Autodesk Fusion 360 part; units mm, degrees
note: some values were not read from the file. Chosen so that the rebuilt part matches the saved one: a direction. Set by a fixed rule: which sketch regions a step uses.
(part 3 of 5)
  spline S34 degree 5 poles (-9.6039, 49.6725) (-9.6022, 49.6779) (-9.5989, 49.6887) (-9.5943, 49.705) (-9.5889, 49.727) (-9.5833, 49.7547) (-9.5784, 49.7827) (-9.574, 49.8108) (-9.5699, 49.8389) (-9.566, 49.8672) (-9.5622, 49.8955) (-9.5587, 49.9238) (-9.5555, 49.9523) (-9.5527, 49.9808) (-9.5502, 50.0094) (-9.5481, 50.0382) (-9.5463, 50.067) (-9.5447, 50.0958) (-9.5434, 50.1247) (-9.5422, 50.1537) (-9.5413, 50.1827) (-9.5406, 50.2117) (-9.5401, 50.2408) (-9.5399, 50.27) (-9.5399, 50.2992) (-9.5401, 50.3285) (-9.5405, 50.3578) (-9.5412, 50.3871) (-9.542, 50.4165) (-9.543, 50.4459) (-9.5442, 50.4754) (-9.5456, 50.5049) (-9.5473, 50.5344) (-9.549, 50.564) (-9.551, 50.5936) (-9.5532, 50.6232) (-9.5556, 50.6529) (-9.5581, 50.6826) (-9.5608, 50.7123) (-9.5637, 50.7421) (-9.5668, 50.7719) (-9.57, 50.8017) (-9.5734, 50.8315) (-9.577, 50.8614) (-9.5807, 50.8913) (-9.5846, 50.9212) (-9.5887, 50.9511) (-9.593, 50.9811) (-9.5974, 51.0111) (-9.6019, 51.0411) (-9.6067, 51.0711) (-9.6116, 51.1012) (-9.6166, 51.1312) (-9.6218, 51.1613) (-9.6272, 51.1914) (-9.6327, 51.2216) (-9.6384, 51.2517) (-9.6442, 51.2818) (-9.6502, 51.312) (-9.6563, 51.3422) (-9.6626, 51.3724) (-9.6691, 51.4026) (-9.6757, 51.4328) (-9.6824, 51.4631) (-9.6893, 51.4933) (-9.6963, 51.5236) (-9.7035, 51.5539) (-9.7108, 51.5841) (-9.7183, 51.6144) (-9.7259, 51.6447) (-9.7337, 51.675) (-9.74, 51.6993) (-9.7448, 51.7175) (-9.748, 51.7296) (-9.7497, 51.7357) knots 0 0 0 0 0 0 0.01428571 0.02857143 0.04285714 0.05714286 0.07142857 0.08571429 0.1 0.11428571 0.12857143 0.14285714 0.15714286 0.17142857 0.18571429 0.2 0.21428571 0.22857143 0.24285714 0.25714286 0.27142857 0.28571429 0.3 0.31428571 0.32857143 0.34285714 0.35714286 0.37142857 0.38571429 0.4 0.41428571 0.42857143 0.44285714 0.45714286 0.47142857 0.48571429 0.5 0.51428571 0.52857143 0.54285714 0.55714286 0.57142857 0.58571429 0.6 0.61428571 0.62857143 0.64285714 0.65714286 0.67142857 0.68571429 0.7 0.71428571 0.72857143 0.74285714 0.75714286 0.77142857 0.78571429 0.8 0.81428571 0.82857143 0.84285714 0.85714286 0.87142857 0.88571429 0.9 0.91428571 0.92857143 0.94285714 0.95714286 0.97142857 0.98571429 1 1 1 1 1 1
  arc A70 (-9.7497, 51.7357) -> (-10.533, 51.9206) centre (-13.5, 37.5997) ccw
  spline S35 degree 5 poles (-10.533, 51.9206) (-10.5372, 51.9159) (-10.5455, 51.9065) (-10.5579, 51.8924) (-10.5744, 51.8735) (-10.5949, 51.8499) (-10.6153, 51.8262) (-10.6355, 51.8024) (-10.6556, 51.7786) (-10.6756, 51.7547) (-10.6954, 51.7308) (-10.7151, 51.7068) (-10.7346, 51.6828) (-10.754, 51.6587) (-10.7733, 51.6346) (-10.7924, 51.6104) (-10.8114, 51.5861) (-10.8303, 51.5618) (-10.849, 51.5375) (-10.8675, 51.513) (-10.8859, 51.4886) (-10.9042, 51.464) (-10.9223, 51.4395) (-10.9403, 51.4148) (-10.9581, 51.3901) (-10.9757, 51.3654) (-10.9933, 51.3406) (-11.0106, 51.3157) (-11.0278, 51.2908) (-11.0448, 51.2659) (-11.0617, 51.2409) (-11.0784, 51.2158) (-11.095, 51.1907) (-11.1114, 51.1655) (-11.1276, 51.1403) (-11.1437, 51.115) (-11.1596, 51.0897) (-11.1753, 51.0643) (-11.1908, 51.0389) (-11.2062, 51.0134) (-11.2214, 50.9879) (-11.2364, 50.9623) (-11.2513, 50.9366) (-11.2659, 50.9109) (-11.2803, 50.8852) (-11.2946, 50.8594) (-11.3087, 50.8335) (-11.3226, 50.8076) (-11.3363, 50.7816) (-11.3498, 50.7556) (-11.363, 50.7296) (-11.3761, 50.7034) (-11.3889, 50.6772) (-11.4015, 50.651) (-11.4139, 50.6247) (-11.426, 50.5983) (-11.4379, 50.5719) (-11.4497, 50.5455) (-11.4612, 50.519) (-11.4724, 50.4924) (-11.4834, 50.4658) (-11.494, 50.4391) (-11.5042, 50.4123) (-11.514, 50.3854) (-11.5236, 50.3585) (-11.5329, 50.3315) (-11.542, 50.3045) (-11.5509, 50.2774) (-11.5595, 50.2503) (-11.5677, 50.2231) (-11.575, 50.1958) (-11.5801, 50.1737) (-11.5833, 50.1571) (-11.5851, 50.1459) (-11.586, 50.1403) knots -1 -1 -1 -1 -1 -1 -0.98571429 -0.97142857 -0.95714286 -0.94285714 -0.92857143 -0.91428571 -0.9 -0.88571429 -0.87142857 -0.85714286 -0.84285714 -0.82857143 -0.81428571 -0.8 -0.78571429 -0.77142857 -0.75714286 -0.74285714 -0.72857143 -0.71428571 -0.7 -0.68571429 -0.67142857 -0.65714286 -0.64285714 -0.62857143 -0.61428571 -0.6 -0.58571429 -0.57142857 -0.55714286 -0.54285714 -0.52857143 -0.51428571 -0.5 -0.48571429 -0.47142857 -0.45714286 -0.44285714 -0.42857143 -0.41428571 -0.4 -0.38571429 -0.37142857 -0.35714286 -0.34285714 -0.32857143 -0.31428571 -0.3 -0.28571429 -0.27142857 -0.25714286 -0.24285714 -0.22857143 -0.21428571 -0.2 -0.18571429 -0.17142857 -0.15714286 -0.14285714 -0.12857143 -0.11428571 -0.1 -0.08571429 -0.07142857 -0.05714286 -0.04285714 -0.02857143 -0.01428571 0 0 0 0 0 0
  line L35 (-11.586, 50.1403) -> (-11.6601, 49.6588)
  arc A71 (-11.7733, 49.5751) -> (-11.6601, 49.6588) centre (-11.759, 49.674) ccw
  arc A72 (-11.7733, 49.5751) -> (-12.7912, 49.6781) centre (-13.5, 37.5997) ccw
  arc A73 (-12.8852, 49.7829) -> (-12.7912, 49.6781) centre (-12.7853, 49.778) ccw
  line L36 (-12.8852, 49.7829) -> (-12.8614, 50.2695)
  spline S36 degree 5 poles (-12.8614, 50.2695) (-12.8611, 50.2751) (-12.8607, 50.2864) (-12.8605, 50.3034) (-12.861, 50.326) (-12.8627, 50.3543) (-12.8652, 50.3825) (-12.8683, 50.4108) (-12.8716, 50.4391) (-12.8751, 50.4674) (-12.8788, 50.4957) (-12.8827, 50.524) (-12.887, 50.5523) (-12.8916, 50.5806) (-12.8967, 50.6089) (-12.902, 50.6372) (-12.9077, 50.6654) (-12.9137, 50.6937) (-12.9199, 50.722) (-12.9263, 50.7502) (-12.9329, 50.7785) (-12.9397, 50.8068) (-12.9468, 50.835) (-12.9541, 50.8632) (-12.9617, 50.8914) (-12.9695, 50.9196) (-12.9775, 50.9478) (-12.9857, 50.976) (-12.9941, 51.0042) (-13.0027, 51.0323) (-13.0115, 51.0605) (-13.0205, 51.0886) (-13.0297, 51.1167) (-13.0391, 51.1448) (-13.0486, 51.1729) (-13.0584, 51.201) (-13.0684, 51.229) (-13.0785, 51.257) (-13.0888, 51.2851) (-13.0993, 51.3131) (-13.11, 51.341) (-13.1208, 51.369) (-13.1318, 51.3969) (-13.143, 51.4249) (-13.1544, 51.4528) (-13.1659, 51.4807) (-13.1776, 51.5085) (-13.1895, 51.5364) (-13.2015, 51.5642) (-13.2137, 51.592) (-13.226, 51.6198) (-13.2385, 51.6475) (-13.2512, 51.6753) (-13.264, 51.703) (-13.277, 51.7307) (-13.2901, 51.7583) (-13.3034, 51.786) (-13.3168, 51.8136) (-13.3304, 51.8412) (-13.3441, 51.8687) (-13.358, 51.8963) (-13.3721, 51.9238) (-13.3862, 51.9513) (-13.4006, 51.9788) (-13.4151, 52.0062) (-13.4297, 52.0336) (-13.4445, 52.061) (-13.4594, 52.0883) (-13.4744, 52.1157) (-13.4896, 52.143) (-13.505, 52.1702) (-13.5173, 52.192) (-13.5267, 52.2084) (-13.533, 52.2192) (-13.5361, 52.2247) knots 0 0 0 0 0 0 0.01428571 0.02857143 0.04285714 0.05714286 0.07142857 0.08571429 0.1 0.11428571 0.12857143 0.14285714 0.15714286 0.17142857 0.18571429 0.2 0.21428571 0.22857143 0.24285714 0.25714286 0.27142857 0.28571429 0.3 0.31428571 0.32857143 0.34285714 0.35714286 0.37142857 0.38571429 0.4 0.41428571 0.42857143 0.44285714 0.45714286 0.47142857 0.48571429 0.5 0.51428571 0.52857143 0.54285714 0.55714286 0.57142857 0.58571429 0.6 0.61428571 0.62857143 0.64285714 0.65714286 0.67142857 0.68571429 0.7 0.71428571 0.72857143 0.74285714 0.75714286 0.77142857 0.78571429 0.8 0.81428571 0.82857143 0.84285714 0.85714286 0.87142857 0.88571429 0.9 0.91428571 0.92857143 0.94285714 0.95714286 0.97142857 0.98571429 1 1 1 1 1 1
  arc A74 (-13.5361, 52.2247) -> (-14.3406, 52.2005) centre (-13.5, 37.5997) ccw
  spline S37 degree 5 poles (-14.3406, 52.2005) (-14.3434, 52.1949) (-14.349, 52.1837) (-14.3574, 52.1668) (-14.3684, 52.1443) (-14.3821, 52.1162) (-14.3957, 52.088) (-14.4091, 52.0598) (-14.4223, 52.0317) (-14.4354, 52.0034) (-14.4484, 51.9752) (-14.4612, 51.9469) (-14.4738, 51.9187) (-14.4863, 51.8904) (-14.4987, 51.8621) (-14.5109, 51.8337) (-14.523, 51.8054) (-14.5349, 51.777) (-14.5466, 51.7487) (-14.5583, 51.7203) (-14.5697, 51.6919) (-14.581, 51.6635) (-14.5921, 51.635) (-14.6031, 51.6066) (-14.6139, 51.5781) (-14.6246, 51.5497) (-14.6351, 51.5212) (-14.6454, 51.4927) (-14.6556, 51.4642) (-14.6656, 51.4357) (-14.6754, 51.4071) (-14.6851, 51.3786) (-14.6946, 51.3501) (-14.7039, 51.3215) (-14.713, 51.2929) (-14.722, 51.2644) (-14.7308, 51.2358) (-14.7394, 51.2072) (-14.7478, 51.1786) (-14.7561, 51.15) (-14.7642, 51.1214) (-14.772, 51.0928) (-14.7797, 51.0642) (-14.7872, 51.0356) (-14.7945, 51.007) (-14.8016, 50.9784) (-14.8085, 50.9497) (-14.8152, 50.9211) (-14.8217, 50.8925) (-14.828, 50.8639) (-14.8341, 50.8353) (-14.8399, 50.8066) (-14.8456, 50.778) (-14.8509, 50.7494) (-14.8561, 50.7208) (-14.861, 50.6922) (-14.8657, 50.6636) (-14.8701, 50.635) (-14.8744, 50.6064) (-14.8784, 50.5779) (-14.8821, 50.5493) (-14.8854, 50.5208) (-14.8883, 50.4923) (-14.8909, 50.4637) (-14.8931, 50.4353) (-14.8951, 50.4068) (-14.8969, 50.3783) (-14.8985, 50.3499) (-14.8999, 50.3215) (-14.9007, 50.2931) (-14.9007, 50.2648) (-14.8999, 50.2422) (-14.8987, 50.2253) (-14.8976, 50.214) (-14.897, 50.2084) knots -1 -1 -1 -1 -1 -1 -0.98571429 -0.97142857 -0.95714286 -0.94285714 -0.92857143 -0.91428571 -0.9 -0.88571429 -0.87142857 -0.85714286 -0.84285714 -0.82857143 -0.81428571 -0.8 -0.78571429 -0.77142857 -0.75714286 -0.74285714 -0.72857143 -0.71428571 -0.7 -0.68571429 -0.67142857 -0.65714286 -0.64285714 -0.62857143 -0.61428571 -0.6 -0.58571429 -0.57142857 -0.55714286 -0.54285714 -0.52857143 -0.51428571 -0.5 -0.48571429 -0.47142857 -0.45714286 -0.44285714 -0.42857143 -0.41428571 -0.4 -0.38571429 -0.37142857 -0.35714286 -0.34285714 -0.32857143 -0.31428571 -0.3 -0.28571429 -0.27142857 -0.25714286 -0.24285714 -0.22857143 -0.21428571 -0.2 -0.18571429 -0.17142857 -0.15714286 -0.14285714 -0.12857143 -0.11428571 -0.1 -0.08571429 -0.07142857 -0.05714286 -0.04285714 -0.02857143 -0.01428571 0 0 0 0 0 0
  line L37 (-14.897, 50.2084) -> (-14.844, 49.7241)
  arc A75 (-14.9315, 49.6139) -> (-14.844, 49.7241) centre (-14.9434, 49.7132) ccw
  arc A76 (-14.9315, 49.6139) -> (-15.9415, 49.45) centre (-13.5, 37.5997) ccw
  arc A77 (-16.0594, 49.5269) -> (-15.9415, 49.45) centre (-15.9617, 49.548) ccw
  line L38 (-16.0594, 49.5269) -> (-16.1623, 50.0031)
  spline S38 degree 5 poles (-16.1623, 50.0031) (-16.1635, 50.0086) (-16.166, 50.0196) (-16.1702, 50.036) (-16.1765, 50.0577) (-16.1855, 50.0846) (-16.1953, 50.1112) (-16.2056, 50.1378) (-16.2161, 50.1642) (-16.2268, 50.1907) (-16.2377, 50.217) (-16.2488, 50.2434) (-16.2602, 50.2696) (-16.2721, 50.2957) (-16.2842, 50.3218) (-16.2968, 50.3477) (-16.3096, 50.3735) (-16.3227, 50.3993) (-16.336, 50.425) (-16.3495, 50.4506) (-16.3632, 50.4762) (-16.3771, 50.5017) (-16.3912, 50.5272) (-16.4056, 50.5526) (-16.4202, 50.5779) (-16.435, 50.6031) (-16.45, 50.6282) (-16.4652, 50.6533) (-16.4806, 50.6784) (-16.4962, 50.7033) (-16.512, 50.7282) (-16.528, 50.7531) (-16.5442, 50.7779) (-16.5605, 50.8026) (-16.577, 50.8272) (-16.5937, 50.8518) (-16.6106, 50.8763) (-16.6276, 50.9008) (-16.6449, 50.9252) (-16.6622, 50.9495) (-16.6798, 50.9738) (-16.6975, 50.998) (-16.7154, 51.0221) (-16.7334, 51.0462) (-16.7516, 51.0702) (-16.7699, 51.0941) (-16.7884, 51.118) (-16.8071, 51.1419) (-16.8259, 51.1656) (-16.8449, 51.1893) (-16.864, 51.213) (-16.8833, 51.2365) (-16.9027, 51.2601) (-16.9222, 51.2835) (-16.9419, 51.3069) (-16.9618, 51.3302) (-16.9817, 51.3535) (-17.0019, 51.3767) (-17.0221, 51.3998) (-17.0425, 51.4229) (-17.0631, 51.4459) (-17.0838, 51.4688) (-17.1046, 51.4917) (-17.1255, 51.5145) (-17.1466, 51.5373) (-17.1678, 51.56) (-17.1892, 51.5826) (-17.2107, 51.6052) (-17.2323, 51.6277) (-17.254, 51.6501) (-17.2759, 51.6725) (-17.2935, 51.6903) (-17.3068, 51.7037) (-17.3156, 51.7126) (-17.3201, 51.717) knots 0 0 0 0 0 0 0.01428571 0.02857143 0.04285714 0.05714286 0.07142857 0.08571429 0.1 0.11428571 0.12857143 0.14285714 0.15714286 0.17142857 0.18571429 0.2 0.21428571 0.22857143 0.24285714 0.25714286 0.27142857 0.28571429 0.3 0.31428571 0.32857143 0.34285714 0.35714286 0.37142857 0.38571429 0.4 0.41428571 0.42857143 0.44285714 0.45714286 0.47142857 0.48571429 0.5 0.51428571 0.52857143 0.54285714 0.55714286 0.57142857 0.58571429 0.6 0.61428571 0.62857143 0.64285714 0.65714286 0.67142857 0.68571429 0.7 0.71428571 0.72857143 0.74285714 0.75714286 0.77142857 0.78571429 0.8 0.81428571 0.82857143 0.84285714 0.85714286 0.87142857 0.88571429 0.9 0.91428571 0.92857143 0.94285714 0.95714286 0.97142857 0.98571429 1 1 1 1 1 1
  arc A78 (-17.3201, 51.717) -> (-18.091, 51.4855) centre (-13.5, 37.5997) ccw
  spline S39 degree 5 poles (-18.091, 51.4855) (-18.0922, 51.4793) (-18.0947, 51.467) (-18.0984, 51.4485) (-18.1033, 51.424) (-18.1092, 51.3932) (-18.115, 51.3625) (-18.1206, 51.3319) (-18.1261, 51.3012) (-18.1315, 51.2705) (-18.1367, 51.2399) (-18.1417, 51.2093) (-18.1467, 51.1787) (-18.1514, 51.1482) (-18.156, 51.1176) (-18.1605, 51.0871) (-18.1648, 51.0566) (-18.169, 51.0261) (-18.173, 50.9957) (-18.1769, 50.9652) (-18.1806, 50.9348) (-18.1841, 50.9045) (-18.1875, 50.8741) (-18.1908, 50.8438) (-18.1938, 50.8135) (-18.1968, 50.7833) (-18.1995, 50.753) (-18.2021, 50.7228) (-18.2046, 50.6927) (-18.2069, 50.6625) (-18.209, 50.6325) (-18.2109, 50.6024) (-18.2127, 50.5724) (-18.2143, 50.5424) (-18.2158, 50.5124) (-18.217, 50.4825) (-18.2181, 50.4526) (-18.2191, 50.4228) (-18.2198, 50.393) (-18.2204, 50.3632) (-18.2208, 50.3335) (-18.221, 50.3038) (-18.221, 50.2742) (-18.2208, 50.2446) (-18.2205, 50.2151) (-18.2199, 50.1856) (-18.2192, 50.1562) (-18.2182, 50.1268) (-18.2171, 50.0975) (-18.2158, 50.0682) (-18.2143, 50.039) (-18.2125, 50.0098) (-18.2105, 49.9807) (-18.2083, 49.9517) (-18.2058, 49.9228) (-18.2032, 49.8939) (-18.2003, 49.865) (-18.1972, 49.8362) (-18.194, 49.8075) (-18.1904, 49.7789) (-18.1866, 49.7504) (-18.1824, 49.7219) (-18.1779, 49.6936) (-18.173, 49.6654) (-18.1677, 49.6373) (-18.1623, 49.6093) (-18.1567, 49.5814) (-18.1509, 49.5535) (-18.1448, 49.5257) (-18.1383, 49.4981) (-18.131, 49.4707) (-18.1243, 49.4491) (-18.1188, 49.4331) (-18.1148, 49.4225) (-18.1127, 49.4172) knots -1 -1 -1 -1 -1 -1 -0.98571429 -0.97142857 -0.95714286 -0.94285714 -0.92857143 -0.91428571 -0.9 -0.88571429 -0.87142857 -0.85714286 -0.84285714 -0.82857143 -0.81428571 -0.8 -0.78571429 -0.77142857 -0.75714286 -0.74285714 -0.72857143 -0.71428571 -0.7 -0.68571429 -0.67142857 -0.65714286 -0.64285714 -0.62857143 -0.61428571 -0.6 -0.58571429 -0.57142857 -0.55714286 -0.54285714 -0.52857143 -0.51428571 -0.5 -0.48571429 -0.47142857 -0.45714286 -0.44285714 -0.42857143 -0.41428571 -0.4 -0.38571429 -0.37142857 -0.35714286 -0.34285714 -0.32857143 -0.31428571 -0.3 -0.28571429 -0.27142857 -0.25714286 -0.24285714 -0.22857143 -0.21428571 -0.2 -0.18571429 -0.17142857 -0.15714286 -0.14285714 -0.12857143 -0.11428571 -0.1 -0.08571429 -0.07142857 -0.05714286 -0.04285714 -0.02857143 -0.01428571 0 0 0 0 0 0
  line L39 (-18.1127, 49.4172) -> (-17.9362, 48.9631)
  arc A79 (-17.9923, 48.834) -> (-17.9362, 48.9631) centre (-18.0294, 48.9269) ccw
  arc A80 (-17.9923, 48.834) -> (-18.9254, 48.4143) centre (-13.5, 37.5997) ccw
  arc A81 (-19.0592, 48.458) -> (-18.9254, 48.4143) centre (-18.9702, 48.5037) ccw
  line L40 (-19.0592, 48.458) -> (-19.2818, 48.8914)
  spline S40 degree 5 poles (-19.2818, 48.8914) (-19.2844, 48.8964) (-19.2897, 48.9064) (-19.298, 48.9212) (-19.3097, 48.9405) (-19.3254, 48.9641) (-19.3417, 48.9873) (-19.3584, 49.0103) (-19.3755, 49.0331) (-19.3926, 49.0559) (-19.41, 49.0786) (-19.4276, 49.1011) (-19.4454, 49.1235) (-19.4636, 49.1457) (-19.4821, 49.1677) (-19.5009, 49.1895) (-19.52, 49.2111) (-19.5393, 49.2326) (-19.5587, 49.254) (-19.5784, 49.2753) (-19.5983, 49.2964) (-19.6183, 49.3175) (-19.6386, 49.3384) (-19.659, 49.3592) (-19.6797, 49.3798) (-19.7005, 49.4004) (-19.7215, 49.4208) (-19.7427, 49.4411) (-19.7641, 49.4613) (-19.7856, 49.4814) (-19.8073, 49.5013) (-19.8292, 49.5212) (-19.8512, 49.5409) (-19.8734, 49.5606) (-19.8957, 49.5801) (-19.9182, 49.5995) (-19.9408, 49.6188) (-19.9636, 49.6381) (-19.9866, 49.6572) (-20.0097, 49.6762) (-20.0329, 49.6951) (-20.0563, 49.7139) (-20.0798, 49.7325) (-20.1034, 49.7511) (-20.1272, 49.7696) (-20.1511, 49.788) (-20.1752, 49.8063) (-20.1994, 49.8245) (-20.2237, 49.8426) (-20.2482, 49.8606) (-20.2727, 49.8784) (-20.2974, 49.8962) (-20.3223, 49.9139) (-20.3472, 49.9315) (-20.3723, 49.949) (-20.3975, 49.9664) (-20.4228, 49.9837) (-20.4483, 50.0009) (-20.4738, 50.018) (-20.4995, 50.035) (-20.5253, 50.0519) (-20.5512, 50.0687) (-20.5773, 50.0854) (-20.6034, 50.102) (-20.6297, 50.1186) (-20.6561, 50.135) (-20.6825, 50.1513) (-20.7091, 50.1675) (-20.7358, 50.1837) (-20.7626, 50.1997) (-20.7896, 50.2157) (-20.8112, 50.2283) (-20.8274, 50.2378) (-20.8383, 50.2441) (-20.8437, 50.2472) knots 0 0 0 0 0 0 0.01428571 0.02857143 0.04285714 0.05714286 0.07142857 0.08571429 0.1 0.11428571 0.12857143 0.14285714 0.15714286 0.17142857 0.18571429 0.2 0.21428571 0.22857143 0.24285714 0.25714286 0.27142857 0.28571429 0.3 0.31428571 0.32857143 0.34285714 0.35714286 0.37142857 0.38571429 0.4 0.41428571 0.42857143 0.44285714 0.45714286 0.47142857 0.48571429 0.5 0.51428571 0.52857143 0.54285714 0.55714286 0.57142857 0.58571429 0.6 0.61428571 0.62857143 0.64285714 0.65714286 0.67142857 0.68571429 0.7 0.71428571 0.72857143 0.74285714 0.75714286 0.77142857 0.78571429 0.8 0.81428571 0.82857143 0.84285714 0.85714286 0.87142857 0.88571429 0.9 0.91428571 0.92857143 0.94285714 0.95714286 0.97142857 0.98571429 1 1 1 1 1 1
  arc A82 (-20.8437, 50.2472) -> (-21.5284, 49.8241) centre (-13.5, 37.5997) ccw
  spline S41 degree 5 poles (-21.5284, 49.8241) (-21.528, 49.8178) (-21.5273, 49.8053) (-21.5261, 49.7865) (-21.5244, 49.7615) (-21.5222, 49.7303) (-21.5198, 49.6991) (-21.5173, 49.668) (-21.5147, 49.637) (-21.5119, 49.606) (-21.509, 49.5751) (-21.506, 49.5442) (-21.5028, 49.5134) (-21.4995, 49.4826) (-21.4961, 49.4519) (-21.4925, 49.4213) (-21.4888, 49.3907) (-21.4849, 49.3602) (-21.4809, 49.3297) (-21.4768, 49.2994) (-21.4725, 49.269) (-21.468, 49.2388) (-21.4635, 49.2086) (-21.4588, 49.1785) (-21.4539, 49.1484) (-21.4489, 49.1184) (-21.4437, 49.0885) (-21.4384, 49.0587) (-21.433, 49.0289) (-21.4274, 48.9992) (-21.4216, 48.9696) (-21.4157, 48.9401) (-21.4097, 48.9106) (-21.4035, 48.8812) (-21.3971, 48.8519) (-21.3906, 48.8227) (-21.3839, 48.7935) (-21.3771, 48.7645) (-21.3701, 48.7355) (-21.363, 48.7066) (-21.3557, 48.6778) (-21.3482, 48.6491) (-21.3405, 48.6204) (-21.3327, 48.5919) (-21.3247, 48.5635) (-21.3166, 48.5352) (-21.3082, 48.5069) (-21.2997, 48.4788) (-21.291, 48.4507) (-21.2822, 48.4228) (-21.2731, 48.395) (-21.2639, 48.3673) (-21.2544, 48.3397) (-21.2448, 48.3122) (-21.2349, 48.2849) (-21.2249, 48.2577) (-21.2146, 48.2306) (-21.2042, 48.2036) (-21.1936, 48.1767) (-21.1828, 48.1499) (-21.1717, 48.1234) (-21.1603, 48.097) (-21.1486, 48.0708) (-21.1366, 48.0448) (-21.1243, 48.0191) (-21.1117, 47.9934) (-21.0991, 47.9679) (-21.0862, 47.9424) (-21.0732, 47.9172) (-21.0597, 47.8922) (-21.0456, 47.8676) (-21.0336, 47.8485) (-21.0241, 47.8345) (-21.0175, 47.8252) (-21.0142, 47.8207) knots -1 -1 -1 -1 -1 -1 -0.98571429 -0.97142857 -0.95714286 -0.94285714 -0.92857143 -0.91428571 -0.9 -0.88571429 -0.87142857 -0.85714286 -0.84285714 -0.82857143 -0.81428571 -0.8 -0.78571429 -0.77142857 -0.75714286 -0.74285714 -0.72857143 -0.71428571 -0.7 -0.68571429 -0.67142857 -0.65714286 -0.64285714 -0.62857143 -0.61428571 -0.6 -0.58571429 -0.57142857 -0.55714286 -0.54285714 -0.52857143 -0.51428571 -0.5 -0.48571429 -0.47142857 -0.45714286 -0.44285714 -0.42857143 -0.41428571 -0.4 -0.38571429 -0.37142857 -0.35714286 -0.34285714 -0.32857143 -0.31428571 -0.3 -0.28571429 -0.27142857 -0.25714286 -0.24285714 -0.22857143 -0.21428571 -0.2 -0.18571429 -0.17142857 -0.15714286 -0.14285714 -0.12857143 -0.11428571 -0.1 -0.08571429 -0.07142857 -0.05714286 -0.04285714 -0.02857143 -0.01428571 0 0 0 0 0 0
  line L41 (-21.0142, 47.8207) -> (-20.7261, 47.4278)
  arc A83 (-20.7469, 47.2886) -> (-20.7261, 47.4278) centre (-20.8068, 47.3686) ccw
  arc A84 (-20.7469, 47.2886) -> (-21.5395, 46.6416) centre (-13.5, 37.5997) ccw
  arc A85 (-21.6801, 46.6492) -> (-21.5395, 46.6416) centre (-21.606, 46.7164) ccw
  line L42 (-21.6801, 46.6492) -> (-22.0073, 47.0102)
  spline S42 degree 5 poles (-22.0073, 47.0102) (-22.0111, 47.0144) (-22.0188, 47.0227) (-22.0306, 47.0348) (-22.047, 47.0504) (-22.0682, 47.0692) (-22.09, 47.0874) (-22.1121, 47.1052) (-22.1344, 47.1229) (-22.1569, 47.1404) (-22.1796, 47.1578) (-22.2024, 47.175) (-22.2254, 47.192) (-22.2487, 47.2088) (-22.2722, 47.2252) (-22.2961, 47.2414) (-22.3201, 47.2574) (-22.3443, 47.2731) (-22.3687, 47.2888) (-22.3932, 47.3042) (-22.4178, 47.3195) (-22.4426, 47.3347) (-22.4676, 47.3496) (-22.4927, 47.3644) (-22.518, 47.379) (-22.5435, 47.3935) (-22.569, 47.4077) (-22.5948, 47.4219) (-22.6206, 47.4358) (-22.6466, 47.4497) (-22.6728, 47.4633) (-22.699, 47.4769) (-22.7254, 47.4902) (-22.7519, 47.5035) (-22.7785, 47.5166) (-22.8053, 47.5295) (-22.8322, 47.5423) (-22.8591, 47.5549) (-22.8862, 47.5675) (-22.9135, 47.5798) (-22.9408, 47.5921) (-22.9682, 47.6042) (-22.9958, 47.6162) (-23.0234, 47.628) (-23.0512, 47.6397) (-23.0791, 47.6513) (-23.107, 47.6627) (-23.1351, 47.674) (-23.1633, 47.6852) (-23.1916, 47.6962) (-23.2199, 47.7071) (-23.2484, 47.7179) (-23.277, 47.7286) (-23.3056, 47.7391) (-23.3344, 47.7495) (-23.3632, 47.7598) (-23.3922, 47.77) (-23.4212, 47.78) (-23.4503, 47.7899) (-23.4795, 47.7997) (-23.5088, 47.8093) (-23.5382, 47.8188) (-23.5677, 47.8282) (-23.5972, 47.8375) (-23.6269, 47.8467) (-23.6566, 47.8557) (-23.6864, 47.8647) (-23.7163, 47.8734) (-23.7462, 47.8821) (-23.7763, 47.8907) (-23.8064, 47.8991) (-23.8306, 47.9058) (-23.8487, 47.9107) (-23.8609, 47.914) (-23.8669, 47.9156) knots 0 0 0 0 0 0 0.01428571 0.02857143 0.04285714 0.05714286 0.07142857 0.08571429 0.1 0.11428571 0.12857143 0.14285714 0.15714286 0.17142857 0.18571429 0.2 0.21428571 0.22857143 0.24285714 0.25714286 0.27142857 0.28571429 0.3 0.31428571 0.32857143 0.34285714 0.35714286 0.37142857 0.38571429 0.4 0.41428571 0.42857143 0.44285714 0.45714286 0.47142857 0.48571429 0.5 0.51428571 0.52857143 0.54285714 0.55714286 0.57142857 0.58571429 0.6 0.61428571 0.62857143 0.64285714 0.65714286 0.67142857 0.68571429 0.7 0.71428571 0.72857143 0.74285714 0.75714286 0.77142857 0.78571429 0.8 0.81428571 0.82857143 0.84285714 0.85714286 0.87142857 0.88571429 0.9 0.91428571 0.92857143 0.94285714 0.95714286 0.97142857 0.98571429 1 1 1 1 1 1
  arc A86 (-23.8669, 47.9156) -> (-24.4188, 47.3296) centre (-13.5, 37.5997) ccw
  spline S43 degree 5 poles (-24.4188, 47.3296) (-24.4168, 47.3237) (-24.4128, 47.3118) (-24.4068, 47.2939) (-24.3987, 47.2702) (-24.3885, 47.2407) (-24.3781, 47.2112) (-24.3677, 47.1818) (-24.3571, 47.1525) (-24.3464, 47.1233) (-24.3356, 47.0941) (-24.3247, 47.0651) (-24.3136, 47.0361) (-24.3025, 47.0073) (-24.2912, 46.9785) (-24.2798, 46.9499) (-24.2683, 46.9213) (-24.2567, 46.8928) (-24.2449, 46.8644) (-24.233, 46.8362) (-24.2211, 46.808) (-24.2089, 46.7799) (-24.1967, 46.7519) (-24.1844, 46.7241) (-24.1719, 46.6963) (-24.1593, 46.6686) (-24.1466, 46.6411) (-24.1337, 46.6136) (-24.1208, 46.5863) (-24.1077, 46.559) (-24.0945, 46.5319) (-24.0811, 46.5049) (-24.0676, 46.478) (-24.054, 46.4512) (-24.0403, 46.4246) (-24.0265, 46.398) (-24.0125, 46.3716) (-23.9983, 46.3453) (-23.9841, 46.3191) (-23.9697, 46.293) (-23.9552, 46.2671) (-23.9405, 46.2413) (-23.9257, 46.2156) (-23.9108, 46.1901) (-23.8957, 46.1647) (-23.8805, 46.1395) (-23.8652, 46.1143) (-23.8497, 46.0894) (-23.834, 46.0645) (-23.8182, 46.0398) (-23.8023, 46.0153) (-23.7862, 45.9909) (-23.7699, 45.9667) (-23.7535, 45.9427) (-23.7369, 45.9189) (-23.7201, 45.8952) (-23.7032, 45.8716) (-23.6862, 45.8482) (-23.669, 45.825) (-23.6516, 45.802) (-23.634, 45.7792) (-23.6162, 45.7567) (-23.5981, 45.7344) (-23.5798, 45.7124) (-23.5612, 45.6907) (-23.5425, 45.6692) (-23.5236, 45.6478) (-23.5046, 45.6265) (-23.4855, 45.6055) (-23.466, 45.5849) (-23.446, 45.5648) (-23.4295, 45.5494) (-23.4166, 45.5383) (-23.4079, 45.5312) (-23.4035, 45.5276) knots -1 -1 -1 -1 -1 -1 -0.98571429 -0.97142857 -0.95714286 -0.94285714 -0.92857143 -0.91428571 -0.9 -0.88571429 -0.87142857 -0.85714286 -0.84285714 -0.82857143 -0.81428571 -0.8 -0.78571429 -0.77142857 -0.75714286 -0.74285714 -0.72857143 -0.71428571 -0.7 -0.68571429 -0.67142857 -0.65714286 -0.64285714 -0.62857143 -0.61428571 -0.6 -0.58571429 -0.57142857 -0.55714286 -0.54285714 -0.52857143 -0.51428571 -0.5 -0.48571429 -0.47142857 -0.45714286 -0.44285714 -0.42857143 -0.41428571 -0.4 -0.38571429 -0.37142857 -0.35714286 -0.34285714 -0.32857143 -0.31428571 -0.3 -0.28571429 -0.27142857 -0.25714286 -0.24285714 -0.22857143 -0.21428571 -0.2 -0.18571429 -0.17142857 -0.15714286 -0.14285714 -0.12857143 -0.11428571 -0.1 -0.08571429 -0.07142857 -0.05714286 -0.04285714 -0.02857143 -0.01428571 0 0 0 0 0 0
  line L43 (-23.4035, 45.5276) -> (-23.0236, 45.2226)
  arc A87 (-23.0076, 45.0828) -> (-23.0236, 45.2226) centre (-23.0862, 45.1446) ccw
  arc A88 (-23.0076, 45.0828) -> (-23.6058, 44.2528) centre (-13.5, 37.5997) ccw
  arc A89 (-23.7435, 44.2237) -> (-23.6058, 44.2528) centre (-23.6893, 44.3077) ccw
  line L44 (-23.7435, 44.2237) -> (-24.153, 44.4877)
  spline S44 degree 5 poles (-24.153, 44.4877) (-24.1578, 44.4907) (-24.1673, 44.4968) (-24.1819, 44.5054) (-24.2018, 44.5163) (-24.2271, 44.5289) (-24.2529, 44.5408) (-24.2789, 44.5523) (-24.305, 44.5636) (-24.3313, 44.5747) (-24.3576, 44.5857) (-24.3841, 44.5964) (-24.4107, 44.6069) (-24.4376, 44.617) (-24.4646, 44.6268) (-24.4918, 44.6363) (-24.5191, 44.6455) (-24.5466, 44.6545) (-24.5742, 44.6632) (-24.6018, 44.6718) (-24.6296, 44.6802) (-24.6575, 44.6884) (-24.6855, 44.6964) (-24.7136, 44.7042) (-24.7418, 44.7118) (-24.7701, 44.7191) (-24.7985, 44.7263) (-24.827, 44.7333) (-24.8556, 44.7401) (-24.8843, 44.7467) (-24.9131, 44.7532) (-24.942, 44.7594) (-24.9709, 44.7655) (-24.9999, 44.7714) (-25.029, 44.7772) (-25.0582, 44.7828) (-25.0875, 44.7882) (-25.1168, 44.7934) (-25.1463, 44.7985) (-25.1758, 44.8034) (-25.2053, 44.8081) (-25.235, 44.8127) (-25.2647, 44.8172) (-25.2944, 44.8214) (-25.3243, 44.8256) (-25.3542, 44.8295) (-25.3842, 44.8333) (-25.4142, 44.837) (-25.4443, 44.8405) (-25.4745, 44.8438) (-25.5047, 44.847) (-25.535, 44.8501) (-25.5654, 44.853) (-25.5958, 44.8557) (-25.6262, 44.8584) (-25.6568, 44.8608) (-25.6873, 44.8631) (-25.718, 44.8653) (-25.7487, 44.8673) (-25.7794, 44.8692) (-25.8102, 44.871) (-25.8411, 44.8726) (-25.872, 44.874) (-25.9029, 44.8753) (-25.9339, 44.8765) (-25.965, 44.8776) (-25.9961, 44.8785) (-26.0272, 44.8792) (-26.0584, 44.8798) (-26.0896, 44.8803) (-26.1209, 44.8807) (-26.146, 44.8808) (-26.1648, 44.8809) (-26.1774, 44.8809) (-26.1836, 44.8809) knots 0 0 0 0 0 0 0.01428571 0.02857143 0.04285714 0.05714286 0.07142857 0.08571429 0.1 0.11428571 0.12857143 0.14285714 0.15714286 0.17142857 0.18571429 0.2 0.21428571 0.22857143 0.24285714 0.25714286 0.27142857 0.28571429 0.3 0.31428571 0.32857143 0.34285714 0.35714286 0.37142857 0.38571429 0.4 0.41428571 0.42857143 0.44285714 0.45714286 0.47142857 0.48571429 0.5 0.51428571 0.52857143 0.54285714 0.55714286 0.57142857 0.58571429 0.6 0.61428571 0.62857143 0.64285714 0.65714286 0.67142857 0.68571429 0.7 0.71428571 0.72857143 0.74285714 0.75714286 0.77142857 0.78571429 0.8 0.81428571 0.82857143 0.84285714 0.85714286 0.87142857 0.88571429 0.9 0.91428571 0.92857143 0.94285714 0.95714286 0.97142857 0.98571429 1 1 1 1 1 1
  arc A90 (-26.1836, 44.8809) -> (-26.565, 44.1721) centre (-13.5, 37.5997) ccw
  spline S45 degree 5 poles (-26.565, 44.1721) (-26.5615, 44.1669) (-26.5546, 44.1564) (-26.5442, 44.1407) (-26.5302, 44.1199) (-26.5127, 44.094) (-26.4951, 44.0682) (-26.4774, 44.0425) (-26.4596, 44.017) (-26.4417, 43.9915) (-26.4237, 43.9662) (-26.4056, 43.9409) (-26.3875, 43.9158) (-26.3692, 43.8909) (-26.3509, 43.866) (-26.3325, 43.8413) (-26.314, 43.8166) (-26.2954, 43.7921) (-26.2767, 43.7678) (-26.2579, 43.7435) (-26.239, 43.7194) (-26.2201, 43.6954) (-26.201, 43.6716) (-26.1819, 43.6478) (-26.1626, 43.6242) (-26.1433, 43.6008) (-26.1239, 43.5775) (-26.1044, 43.5543) (-26.0848, 43.5312) (-26.0651, 43.5083) (-26.0453, 43.4855) (-26.0254, 43.4629) (-26.0054, 43.4404) (-25.9854, 43.418) (-25.9652, 43.3958) (-25.9449, 43.3738) (-25.9246, 43.3519) (-25.9041, 43.3301) (-25.8836, 43.3085) (-25.863, 43.2871) (-25.8422, 43.2658) (-25.8214, 43.2446) (-25.8005, 43.2237) (-25.7794, 43.2029) (-25.7583, 43.1823) (-25.7371, 43.1618) (-25.7157, 43.1415) (-25.6943, 43.1214) (-25.6728, 43.1015) (-25.6511, 43.0817) (-25.6294, 43.0621) (-25.6075, 43.0427) (-25.5855, 43.0236) (-25.5634, 43.0046) (-25.5412, 42.9859) (-25.5189, 42.9673) (-25.4965, 42.949) (-25.474, 42.9308) (-25.4514, 42.9128) (-25.4286, 42.8951) (-25.4057, 42.8776) (-25.3827, 42.8605) (-25.3594, 42.8437) (-25.336, 42.8272) (-25.3125, 42.811) (-25.2888, 42.795) (-25.2651, 42.7793) (-25.2412, 42.7636) (-25.2173, 42.7483) (-25.1932, 42.7334) (-25.1687, 42.7192) (-25.1487, 42.7086) (-25.1334, 42.7012) (-25.1231, 42.6965) (-25.1179, 42.6943) knots -1 -1 -1 -1 -1 -1 -0.98571429 -0.97142857 -0.95714286 -0.94285714 -0.92857143 -0.91428571 -0.9 -0.88571429 -0.87142857 -0.85714286 -0.84285714 -0.82857143 -0.81428571 -0.8 -0.78571429 -0.77142857 -0.75714286 -0.74285714 -0.72857143 -0.71428571 -0.7 -0.68571429 -0.67142857 -0.65714286 -0.64285714 -0.62857143 -0.61428571 -0.6 -0.58571429 -0.57142857 -0.55714286 -0.54285714 -0.52857143 -0.51428571 -0.5 -0.48571429 -0.47142857 -0.45714286 -0.44285714 -0.42857143 -0.41428571 -0.4 -0.38571429 -0.37142857 -0.35714286 -0.34285714 -0.32857143 -0.31428571 -0.3 -0.28571429 -0.27142857 -0.25714286 -0.24285714 -0.22857143 -0.21428571 -0.2 -0.18571429 -0.17142857 -0.15714286 -0.14285714 -0.12857143 -0.11428571 -0.1 -0.08571429 -0.07142857 -0.05714286 -0.04285714 -0.02857143 -0.01428571 0 0 0 0 0 0
  line L45 (-25.1179, 42.6943) -> (-24.672, 42.498)
  arc A91 (-24.6204, 42.3671) -> (-24.672, 42.498) centre (-24.7123, 42.4065) ccw
  arc A92 (-24.6204, 42.3671) -> (-24.9834, 41.4105) centre (-13.5, 37.5997) ccw
  arc A93 (-25.1089, 41.3468) -> (-24.9834, 41.4105) centre (-25.0783, 41.442) ccw
  line L46 (-25.1089, 41.3468) -> (-25.5728, 41.4958)
  spline S46 degree 5 poles (-25.5728, 41.4958) (-25.5781, 41.4975) (-25.589, 41.5008) (-25.6053, 41.5054) (-25.6272, 41.5108) (-25.655, 41.5164) (-25.683, 41.5213) (-25.711, 41.5257) (-25.7392, 41.5298) (-25.7675, 41.5337) (-25.7958, 41.5375) (-25.8241, 41.541) (-25.8526, 41.5442) (-25.8811, 41.5471) (-25.9097, 41.5495) (-25.9384, 41.5516) (-25.9672, 41.5535) (-25.9961, 41.555) (-26.025, 41.5563) (-26.054, 41.5575) (-26.083, 41.5584) (-26.112, 41.5591) (-26.1411, 41.5596) (-26.1703, 41.5598) (-26.1995, 41.5598) (-26.2287, 41.5596) (-26.258, 41.5592) (-26.2874, 41.5586) (-26.3168, 41.5577) (-26.3462, 41.5567) (-26.3757, 41.5555) (-26.4051, 41.5541) (-26.4347, 41.5525) (-26.4643, 41.5507) (-26.4939, 41.5487) (-26.5235, 41.5465) (-26.5532, 41.5442) (-26.5829, 41.5416) (-26.6126, 41.5389) (-26.6424, 41.536) (-26.6721, 41.533) (-26.702, 41.5297) (-26.7318, 41.5263) (-26.7617, 41.5227) (-26.7916, 41.519) (-26.8215, 41.5151) (-26.8514, 41.511) (-26.8814, 41.5068) (-26.9114, 41.5023) (-26.9414, 41.4978) (-26.9714, 41.493) (-27.0015, 41.4881) (-27.0315, 41.4831) (-27.0616, 41.4779) (-27.0917, 41.4725) (-27.1218, 41.467) (-27.152, 41.4613) (-27.1821, 41.4555) (-27.2123, 41.4495) (-27.2425, 41.4434) (-27.2727, 41.4371) (-27.3029, 41.4306) (-27.3331, 41.4241) (-27.3634, 41.4173) (-27.3936, 41.4104) (-27.4239, 41.4034) (-27.4541, 41.3962) (-27.4844, 41.3889) (-27.5147, 41.3814) (-27.545, 41.3738) (-27.5753, 41.366) (-27.5996, 41.3597) (-27.6178, 41.3549) (-27.6299, 41.3517) (-27.636, 41.3501) knots 0 0 0 0 0 0 0.01428571 0.02857143 0.04285714 0.05714286 0.07142857 0.08571429 0.1 0.11428571 0.12857143 0.14285714 0.15714286 0.17142857 0.18571429 0.2 0.21428571 0.22857143 0.24285714 0.25714286 0.27142857 0.28571429 0.3 0.31428571 0.32857143 0.34285714 0.35714286 0.37142857 0.38571429 0.4 0.41428571 0.42857143 0.44285714 0.45714286 0.47142857 0.48571429 0.5 0.51428571 0.52857143 0.54285714 0.55714286 0.57142857 0.58571429 0.6 0.61428571 0.62857143 0.64285714 0.65714286 0.67142857 0.68571429 0.7 0.71428571 0.72857143 0.74285714 0.75714286 0.77142857 0.78571429 0.8 0.81428571 0.82857143 0.84285714 0.85714286 0.87142857 0.88571429 0.9 0.91428571 0.92857143 0.94285714 0.95714286 0.97142857 0.98571429 1 1 1 1 1 1
  arc A94 (-27.636, 41.3501) -> (-27.8209, 40.5667) centre (-13.5, 37.5997) ccw
  spline S47 degree 5 poles (-27.8209, 40.5667) (-27.8162, 40.5625) (-27.8068, 40.5542) (-27.7927, 40.5418) (-27.7738, 40.5253) (-27.7501, 40.5048) (-27.7264, 40.4844) (-27.7027, 40.4642) (-27.6789, 40.4441) (-27.655, 40.4241) (-27.6311, 40.4043) (-27.6071, 40.3846) (-27.5831, 40.3651) (-27.559, 40.3457) (-27.5349, 40.3264) (-27.5107, 40.3073) (-27.4864, 40.2883) (-27.4621, 40.2695) (-27.4377, 40.2508) (-27.4133, 40.2322) (-27.3888, 40.2138) (-27.3643, 40.1955) (-27.3397, 40.1774) (-27.3151, 40.1594) (-27.2904, 40.1416) (-27.2657, 40.124) (-27.2409, 40.1065) (-27.216, 40.0891) (-27.1911, 40.0719) (-27.1662, 40.0549) (-27.1412, 40.038) (-27.1161, 40.0213) (-27.091, 40.0047) (-27.0658, 39.9883) (-27.0406, 39.9721) (-27.0153, 39.956) (-26.99, 39.9401) (-26.9646, 39.9244) (-26.9392, 39.9089) (-26.9137, 39.8935) (-26.8882, 39.8783) (-26.8626, 39.8633) (-26.8369, 39.8485) (-26.8112, 39.8338) (-26.7855, 39.8194) (-26.7597, 39.8051) (-26.7338, 39.791) (-26.7079, 39.7771) (-26.6819, 39.7634) (-26.6559, 39.75) (-26.6298, 39.7367) (-26.6037, 39.7236) (-26.5775, 39.7108) (-26.5513, 39.6982) (-26.525, 39.6859) (-26.4986, 39.6737) (-26.4722, 39.6618) (-26.4458, 39.6501) (-26.4193, 39.6385) (-26.3927, 39.6273) (-26.3661, 39.6163) (-26.3394, 39.6057) (-26.3126, 39.5955) (-26.2857, 39.5857) (-26.2587, 39.5761) (-26.2318, 39.5668) (-26.2047, 39.5577) (-26.1777, 39.5488) (-26.1506, 39.5402) (-26.1234, 39.532) (-26.0961, 39.5247) (-26.074, 39.5196) (-26.0574, 39.5164) (-26.0462, 39.5146) (-26.0406, 39.5137) knots -1 -1 -1 -1 -1 -1 -0.98571429 -0.97142857 -0.95714286 -0.94285714 -0.92857143 -0.91428571 -0.9 -0.88571429 -0.87142857 -0.85714286 -0.84285714 -0.82857143 -0.81428571 -0.8 -0.78571429 -0.77142857 -0.75714286 -0.74285714 -0.72857143 -0.71428571 -0.7 -0.68571429 -0.67142857 -0.65714286 -0.64285714 -0.62857143 -0.61428571 -0.6 -0.58571429 -0.57142857 -0.55714286 -0.54285714 -0.52857143 -0.51428571 -0.5 -0.48571429 -0.47142857 -0.45714286 -0.44285714 -0.42857143 -0.41428571 -0.4 -0.38571429 -0.37142857 -0.35714286 -0.34285714 -0.32857143 -0.31428571 -0.3 -0.28571429 -0.27142857 -0.25714286 -0.24285714 -0.22857143 -0.21428571 -0.2 -0.18571429 -0.17142857 -0.15714286 -0.14285714 -0.12857143 -0.11428571 -0.1 -0.08571429 -0.07142857 -0.05714286 -0.04285714 -0.02857143 -0.01428571 0 0 0 0 0 0
  line L47 (-26.0406, 39.5137) -> (-25.5591, 39.4396)
  arc A95 (-25.4753, 39.3265) -> (-25.5591, 39.4396) centre (-25.5743, 39.3407) ccw
  circle A96 centre (-13.5, 37.5997) radius 1.5
sketch "Sketch4 (2)" plane through (-39.3468, 6.9151, 3) normal (0, 0, 1) x (-0.495736, -0.868473, 0) in component "Spur Gear (24 teeth)"
  line L0 (-9.5, 37.5997) -> (-9.5, 68.5997)
  arc A0 (-9.5, 68.5997) -> (-17.5, 68.5997) centre (-13.5, 68.5997) ccw
  line L1 (-17.5, 68.5997) -> (-17.5, 37.5997)
  arc A1 (-17.5, 37.5997) -> (-9.5, 37.5997) centre (-13.5, 37.5997) ccw
  line L2 (-13.5, 37.5997) -> (-13.5, 68.5997) construction
  circle A2 centre (-13.5, 68.5997) radius 1.5
  circle A3 centre (-13.5, 37.5997) radius 1.5
  dimension "d62" = 31
  dimension "d63" = 8
  dimension "d64" = 3
  constraint tangent L0 A0
  constraint tangent A0 L1
  constraint parallel L0 L1
  constraint tangent L1 A1
  constraint tangent L0 A1
  constraint vertical L2
  constraint concentric A0 A2
  measures "d62" distance of A1.centre A0.centre
  measures "d63" diameter of A0
  measures "d64" diameter of A2
extrude "Extrude3" add sketch "Sketch4 (2)" against normal blind 3 bodies 4 in component "Spur Gear (24 teeth)"
ref_plane "WorkPlane1" through (0, 32.7497, 1.5) normal (-1, 0, 0) x (0, -1, 0)
mirror "MirrorComponent1" about plane through (0, 0, 0) normal (0, 0, 1) of bodies 2 makes body 5 in component "Conecting Rod"
mirror "MirrorComponent1'" about plane through (0, 0, 0) normal (0, 0, 1) of bodies 1 makes body 6 in component "Gripper"
sketch "Sketch5" plane through (0, 0, 0) normal (1, 0, 0) x (0, 0, -1)
  line L0 (62.9419, 58.0899) -> (65.4419, 58.0899)
  line L1 (65.4419, 58.0899) -> (65.4419, 47.0899)
  line L2 (62.9419, 57.0899) -> (62.9419, 58.0899)
  line L3 (62.9419, 57.0899) -> (63.9419, 57.0899)
  line L4 (63.9419, 57.0899) -> (63.9419, 48.0899)
  line L5 (63.9419, 48.0899) -> (62.9419, 48.0899)
  line L6 (62.9419, 48.0899) -> (62.9419, 47.0899)
  line L7 (62.9419, 47.0899) -> (65.4419, 47.0899)
  dimension "d133" = 1
  dimension "d134" = 2.5
  dimension "d135" = 11
  dimension "d136" = 1.5
  dimension "d137" = 1
  dimension "d138" = 2.5
  constraint perpendicular L0 L1
  constraint vertical L2
  constraint perpendicular L2 L3
  constraint perpendicular L3 L4
  constraint perpendicular L2 L5
  constraint perpendicular L5 L6
  constraint perpendicular L1 L7
  constraint coincident L1.end L7.end
  measures "d133" distance of L0.start L2.start
  measures "d134" distance of L0.start L0.end
  measures "d135" distance of L0.end L1.end
  measures "d136" distance of L1 L4
  measures "d137" distance of L5 L7
  measures "d138" distance of L6.end L1.end
revolve "Revolve1" add sketch "Sketch5" angle 360 about axis through (0, 58.0899, -65.4419) along (0, -1, 0) separate body makes body 7 in component "Eye shape "
sketch "Sketch1 (4)" plane through (0, 0, 0) normal (0, 0, 1) x (1, 0, 0) in component "Spur Gear (12 teeth)"
  circle A0 centre (0, 0) radius 5.2292
  circle A1 centre (0, 0) radius 1.5
extrude "Extrude1''''" add sketch "Sketch1 (4)" along normal blind 6 separate body makes body 8 in component "Spur Gear (12 teeth)"
sketch "Sketch2 (3)" plane through (0, 0, 0) normal (0, 0, 1) x (1, 0, 0) in component "Spur Gear (12 teeth)"
  spline S0 degree 5 poles (6.1362, -0.9011) (6.1405, -0.9017) (6.1493, -0.9028) (6.1624, -0.9041) (6.18, -0.9051) (6.202, -0.9052) (6.2242, -0.9045) (6.2464, -0.9033) (6.2686, -0.9019) (6.2909, -0.9002) (6.3132, -0.8984) (6.3355, -0.8963) (6.3578, -0.8939) (6.3802, -0.8912) (6.4026, -0.888) (6.425, -0.8845) (6.4474, -0.8806) (6.4699, -0.8765) (6.4923, -0.8722) (6.5148, -0.8676) (6.5373, -0.8629) (6.5598, -0.8579) (6.5822, -0.8526) (6.6047, -0.8471) (6.6272, -0.8414) (6.6497, -0.8354) (6.6722, -0.8292) (6.6947, -0.8228) (6.7172, -0.8162) (6.7397, -0.8093) (6.7622, -0.8023) (6.7847, -0.795) (6.8072, -0.7876) (6.8297, -0.7799) (6.8521, -0.7721) (6.8746, -0.764) (6.8971, -0.7558) (6.9195, -0.7474) (6.9419, -0.7387) (6.9644, -0.7299) (6.9868, -0.7209) (7.0092, -0.7117) (7.0315, -0.7023) (7.0539, -0.6928) (7.0763, -0.683) (7.0986, -0.6731) (7.1209, -0.663) (7.1432, -0.6527) (7.1655, -0.6423) (7.1877, -0.6317) (7.21, -0.6209) (7.2322, -0.6099) (7.2544, -0.5988) (7.2765, -0.5874) (7.2987, -0.576) (7.3208, -0.5643) (7.3429, -0.5525) (7.365, -0.5405) (7.387, -0.5284) (7.409, -0.516) (7.431, -0.5036) (7.453, -0.4909) (7.4749, -0.4781) (7.4968, -0.4652) (7.5187, -0.452) (7.5405, -0.4388) (7.5623, -0.4253) (7.5841, -0.4117) (7.6058, -0.398) (7.6275, -0.3841) (7.6492, -0.37) (7.6665, -0.3586) (7.6795, -0.35) (7.6881, -0.3443) (7.6924, -0.3414) knots 0 0 0 0 0 0 0.01428571 0.02857143 0.04285714 0.05714286 0.07142857 0.08571429 0.1 0.11428571 0.12857143 0.14285714 0.15714286 0.17142857 0.18571429 0.2 0.21428571 0.22857143 0.24285714 0.25714286 0.27142857 0.28571429 0.3 0.31428571 0.32857143 0.34285714 0.35714286 0.37142857 0.38571429 0.4 0.41428571 0.42857143 0.44285714 0.45714286 0.47142857 0.48571429 0.5 0.51428571 0.52857143 0.54285714 0.55714286 0.57142857 0.58571429 0.6 0.61428571 0.62857143 0.64285714 0.65714286 0.67142857 0.68571429 0.7 0.71428571 0.72857143 0.74285714 0.75714286 0.77142857 0.78571429 0.8 0.81428571 0.82857143 0.84285714 0.85714286 0.87142857 0.88571429 0.9 0.91428571 0.92857143 0.94285714 0.95714286 0.97142857 0.98571429 1 1 1 1 1 1
  spline S1 degree 5 poles (6.1362, 0.9011) (6.1405, 0.9017) (6.1493, 0.9028) (6.1624, 0.9041) (6.18, 0.9051) (6.202, 0.9052) (6.2242, 0.9045) (6.2464, 0.9033) (6.2686, 0.9019) (6.2909, 0.9002) (6.3132, 0.8984) (6.3355, 0.8963) (6.3578, 0.8939) (6.3802, 0.8912) (6.4026, 0.888) (6.425, 0.8845) (6.4474, 0.8806) (6.4699, 0.8765) (6.4923, 0.8722) (6.5148, 0.8676) (6.5373, 0.8629) (6.5598, 0.8579) (6.5822, 0.8526) (6.6047, 0.8471) (6.6272, 0.8414) (6.6497, 0.8354) (6.6722, 0.8292) (6.6947, 0.8228) (6.7172, 0.8162) (6.7397, 0.8093) (6.7622, 0.8023) (6.7847, 0.795) (6.8072, 0.7876) (6.8297, 0.7799) (6.8521, 0.7721) (6.8746, 0.764) (6.8971, 0.7558) (6.9195, 0.7474) (6.9419, 0.7387) (6.9644, 0.7299) (6.9868, 0.7209) (7.0092, 0.7117) (7.0315, 0.7023) (7.0539, 0.6928) (7.0763, 0.683) (7.0986, 0.6731) (7.1209, 0.663) (7.1432, 0.6527) (7.1655, 0.6423) (7.1877, 0.6317) (7.21, 0.6209) (7.2322, 0.6099) (7.2544, 0.5988) (7.2765, 0.5874) (7.2987, 0.576) (7.3208, 0.5643) (7.3429, 0.5525) (7.365, 0.5405) (7.387, 0.5284) (7.409, 0.516) (7.431, 0.5036) (7.453, 0.4909) (7.4749, 0.4781) (7.4968, 0.4652) (7.5187, 0.452) (7.5405, 0.4388) (7.5623, 0.4253) (7.5841, 0.4117) (7.6058, 0.398) (7.6275, 0.3841) (7.6492, 0.37) (7.6665, 0.3586) (7.6795, 0.35) (7.6881, 0.3443) (7.6924, 0.3414) knots 0 0 0 0 0 0 0.01428571 0.02857143 0.04285714 0.05714286 0.07142857 0.08571429 0.1 0.11428571 0.12857143 0.14285714 0.15714286 0.17142857 0.18571429 0.2 0.21428571 0.22857143 0.24285714 0.25714286 0.27142857 0.28571429 0.3 0.31428571 0.32857143 0.34285714 0.35714286 0.37142857 0.38571429 0.4 0.41428571 0.42857143 0.44285714 0.45714286 0.47142857 0.48571429 0.5 0.51428571 0.52857143 0.54285714 0.55714286 0.57142857 0.58571429 0.6 0.61428571 0.62857143 0.64285714 0.65714286 0.67142857 0.68571429 0.7 0.71428571 0.72857143 0.74285714 0.75714286 0.77142857 0.78571429 0.8 0.81428571 0.82857143 0.84285714 0.85714286 0.87142857 0.88571429 0.9 0.91428571 0.92857143 0.94285714 0.95714286 0.97142857 0.98571429 1 1 1 1 1 1
  arc A0 (7.6924, -0.3414) -> (7.6924, 0.3414) centre (0, 0) ccw
  line L0 (5.1638, -0.7597) -> (6.1362, -0.9011)
  line L1 (5.1638, 0.7597) -> (6.1362, 0.9011)
  line L2 (5.1638, -0.7597) -> (5.1638, 0.7597)
  point P0 (6.244, -0.9034)
  point P1 (6.3533, -0.8944)
  point P2 (6.4637, -0.8776)
  point P3 (6.5747, -0.8543)
  point P4 (6.6863, -0.8252)
  point P5 (6.7982, -0.7906)
  point P6 (6.9103, -0.7508)
  point P7 (7.0226, -0.7061)
  point P8 (7.1348, -0.6566)
  point P9 (7.247, -0.6024)
  point P10 (7.3589, -0.5438)
  point P11 (7.4705, -0.4806)
  point P12 (7.5817, -0.4132)
  point P13 (6.244, 0.9034)
  point P14 (6.3533, 0.8944)
  point P15 (6.4637, 0.8776)
  point P16 (6.5747, 0.8543)
  point P17 (6.6863, 0.8252)
  point P18 (6.7982, 0.7906)
  point P19 (6.9103, 0.7508)
  point P20 (7.0226, 0.7061)
  point P21 (7.1348, 0.6566)
  point P22 (7.247, 0.6024)
  point P23 (7.3589, 0.5438)
  point P24 (7.4705, 0.4806)
  point P25 (7.5817, 0.4132)
extrude "Extrude2''" add sketch "Sketch2 (3)" along normal blind 6 bodies 8 in component "Spur Gear (12 teeth)"
fillet "Fillet1'" radius 0.1 2 edges at (5.1735, -0.7611, 3) (5.1735, 0.7611, 3) on bodies 8 in component "Spur Gear (12 teeth)"
pattern_circular "C-Pattern1'" count 12 over 360 about axis through (0, 0, 0) along (0, 0, 1) of "Extrude2''", "Fillet1'" in component "Spur Gear (12 teeth)"
sketch "Sketch3 (3)" plane through (0, 0, 0) normal (0, 0, 1) x (1, 0, 0) in component "Spur Gear (12 teeth)"
  circle A0 centre (0, 0) radius 6.6 construction